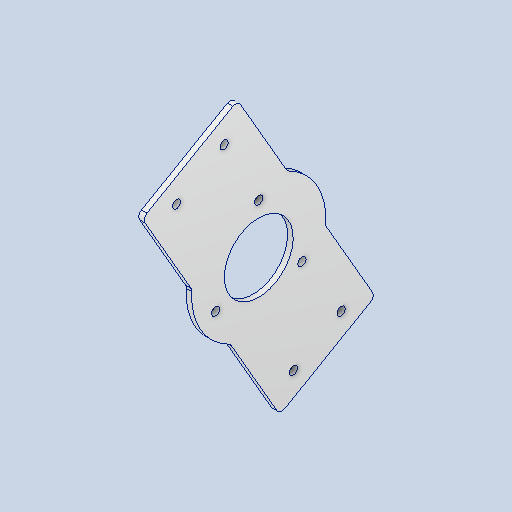
# Autodesk Inventor part: hand-grab-v3-Plate-ASP_F
Saved by Autodesk Inventor 2025.1 (Build 291241000, 241)
## iProperties
Created: 2024-11-30
Part Number: hand-grab-v3-Plate-ASP_F
Material: アルミニウム 6061
Document SubType Name: Modeling
Designer: haruy
Density: 2.7 g/cm^3
Appearance: アルミニウム - フラット
Author: haruy
Autodesk Inventor part; units mm, degrees
ref_plane "YZ Plane" through (0, 0, 0) normal (1, 0, 0) x (0, 1, 0)
ref_plane "XZ Plane" through (0, 0, 0) normal (0, 1, 0) x (-1, 0, 0)
ref_plane "XY Plane" through (0, 0, 0) normal (0, 0, 1) x (1, 0, 0)
sketch "スケッチ1" plane through (0, 0, 0) normal (1, 0, 0) x (0, 1, 0)
  circle A0 centre (73.7666, 7.1685) radius 120
  line L0 (73.7666, 7.1685) -> (-257.6959, 7.1685) construction
  line L1 (141.2666, -109.745) -> (-61.2334, 7.1685)
  circle A1 centre (73.7666, 7.1685) radius 5
  line L2 (73.7666, 7.1685) -> (141.2666, 124.0819) construction
  line L3 (73.7666, 7.1685) -> (141.2666, -109.745) construction
  line L4 (73.7666, 7.1685) -> (-61.2334, 7.1685)
  line L5 (90.8025, 44.6755) -> (85.8025, 36.0153) construction
  line L6 (85.8025, 36.0153) -> (89.2666, 34.0153) construction
  line L7 (89.2666, 34.0153) -> (94.2666, 42.6755) construction
  line L8 (94.2666, 42.6755) -> (90.8025, 44.6755)
  line L9 (94.2666, 42.6755) -> (89.2666, 34.0153) construction
  line L10 (89.2666, 34.0153) -> (92.7307, 32.0153) construction
  line L11 (92.7307, 32.0153) -> (97.7307, 40.6755) construction
  line L12 (97.7307, 40.6755) -> (94.2666, 42.6755)
  line L13 (88.3025, 40.3454) -> (95.2307, 36.3454) construction
  circle A2 centre (73.7666, 7.1685) radius 2.65 construction
  line L14 (90.586, 44.8005) -> (84.086, 33.5422) construction
  line L15 (84.086, 33.5422) -> (79.7559, 36.0422) construction
  line L16 (79.7559, 36.0422) -> (86.2559, 47.3005) construction
  line L17 (86.2559, 47.3005) -> (90.586, 44.8005)
  line L18 (97.9473, 40.5505) -> (91.4473, 29.2922) construction
  line L19 (91.4473, 29.2922) -> (95.7774, 26.7922) construction
  line L20 (95.7774, 26.7922) -> (102.2774, 38.0505) construction
  line L21 (102.2774, 38.0505) -> (97.9473, 40.5505)
  circle A3 centre (73.7666, 7.1685) radius 28.3207 construction
  line L22 (32.7666, 16.4185) -> (32.7666, 11.4185)
  line L23 (32.7666, 11.4185) -> (45.7666, 11.4185) construction
  line L24 (45.7666, 16.4185) -> (32.7666, 16.4185) construction
  line L25 (45.7666, 11.4185) -> (45.7666, 16.4185)
  line L26 (32.7666, 2.9185) -> (45.7666, 2.9185) construction
  line L27 (32.7666, -2.0815) -> (32.7666, 2.9185)
  line L28 (45.7666, -2.0815) -> (32.7666, -2.0815) construction
  line L29 (45.7666, 2.9185) -> (45.7666, -2.0815)
  line L30 (86.2559, -32.9636) -> (90.586, -30.4636)
  line L31 (90.586, -30.4636) -> (84.086, -19.2052) construction
  line L32 (79.7559, -21.7052) -> (86.2559, -32.9636) construction
  line L33 (84.086, -19.2052) -> (79.7559, -21.7052) construction
  line L34 (97.9473, -26.2136) -> (91.4473, -14.9552) construction
  line L35 (102.2774, -23.7136) -> (97.9473, -26.2136)
  line L36 (95.7774, -12.4552) -> (102.2774, -23.7136) construction
  line L37 (91.4473, -14.9552) -> (95.7774, -12.4552) construction
  line L38 (79.7559, 36.0422) -> (79.1397, 34.9748)
  line L39 (95.7774, 26.7922) -> (95.1611, 25.7248) construction
  line L40 (45.7666, 16.4185) -> (46.9991, 16.4185)
  line L41 (45.7666, -2.0815) -> (46.9991, -2.0815)
  line L42 (79.7559, -21.7052) -> (75.9601, -15.1307) construction
  line L43 (95.7774, -12.4552) -> (95.1611, -11.3879) construction
  line L44 (87.3775, 38.7432) -> (77.3775, 21.4227) construction
  line L45 (77.3775, 21.4227) -> (72.1814, 24.4227) construction
  line L46 (72.1814, 24.4227) -> (82.1814, 41.7432) construction
  line L47 (82.1814, 41.7432) -> (87.3775, 38.7432)
  circle A4 centre (77.2795, 27.2529) radius 1.5
  circle A5 centre (82.2795, 35.9131) radius 1.5
  circle A6 centre (89.4038, 20.2529) radius 1.5
  circle A7 centre (94.4038, 28.9131) radius 1.5
  circle A8 centre (44.6166, 14.1685) radius 1.5
  circle A9 centre (54.6166, 14.1685) radius 1.5
  circle A10 centre (54.6166, 0.1685) radius 1.5
  circle A11 centre (44.6166, 0.1685) radius 1.5
  circle A12 centre (82.2795, -21.5762) radius 1.5
  circle A13 centre (77.2795, -12.9159) radius 1.5
  circle A14 centre (89.4038, -5.9159) radius 1.5
  circle A15 centre (94.4038, -14.5762) radius 1.5
  line L48 (74.7795, 22.9227) -> (87.3775, 38.7432) construction
  circle A16 centre (73.7666, 7.1685) radius 34.3835
  line L49 (65.7666, 54.1685) -> (-114.2334, 54.1685) construction
  line L50 (-114.2334, 54.1685) -> (-114.2334, 39.1685)
  line L51 (-114.2334, 39.1685) -> (65.7666, 39.1685) construction
  line L52 (65.7666, 39.1685) -> (65.7666, 54.1685) construction
  circle A17 centre (55.7666, 46.6685) radius 1.5 construction
  circle A18 centre (45.7666, 46.6685) radius 1.5 construction
  line L53 (39.3832, 54.1685) -> (39.3832, 7.1685) construction
  line L54 (65.7666, 54.1685) -> (93.0867, 35.6107) construction
  line L55 (39.3832, -39.8315) -> (39.3832, 7.1685) construction
  line L56 (65.7666, -39.8315) -> (93.0867, -21.2737) construction
  line L57 (65.7666, -39.8315) -> (-114.2334, -39.8315) construction
  line L58 (-114.2334, -24.8315) -> (65.7666, -24.8315) construction
  circle A19 centre (45.7666, -32.3315) radius 1.5 construction
  circle A20 centre (55.7666, -32.3315) radius 1.5 construction
  line L59 (73.7666, 7.1685) -> (56.5749, 36.9454)
  line L60 (65.2352, 41.9454) -> (47.9147, 31.9454)
  line L61 (47.9147, 31.9454) -> (52.9147, 23.2852)
  line L62 (52.9147, 23.2852) -> (70.2352, 33.2852)
  line L63 (70.2352, 33.2852) -> (65.2352, 41.9454)
  circle A21 centre (63.405, 35.1153) radius 1.5
  circle A22 centre (54.7448, 30.1153) radius 1.5
  circle A23 centre (54.7448, -15.7784) radius 1.5
  circle A24 centre (63.405, -20.7784) radius 1.5
  circle A25 centre (103.1501, 2.1685) radius 1.5
  circle A26 centre (103.1501, 12.1685) radius 1.5
  circle A27 centre (73.7666, 7.1685) radius 193.5
  line L64 (-119.0981, 22.835) -> (156.6314, 182.0275)
  line L65 (73.7666, 7.1685) -> (13.7666, 111.0915)
  line L66 (73.7666, 7.1685) -> (73.7666, 200.6685)
  line L67 (127.0679, 14.848) -> (25.5679, 190.6511)
  line L68 (25.5679, 190.6511) -> (12.5775, 183.1511)
  line L69 (12.5775, 183.1511) -> (114.0775, 7.348)
  line L70 (114.0775, 7.348) -> (127.0679, 14.848)
  circle A28 centre (51.8227, 130.1764) radius 1.5
  circle A29 centre (22.8227, 180.4059) radius 1.5
  circle A30 centre (64.6999, 22.8725) radius 1.5
  circle A31 centre (73.7666, 7.1685) radius 12.5
  circle A32 centre (64.6999, -8.5356) radius 1.5
  circle A33 centre (91.9001, 7.1685) radius 1.5
  circle A34 centre (115.5727, 19.7582) radius 1.5
  circle A35 centre (105.5727, 37.0787) radius 1.5
  circle A36 centre (73.7666, 7.1685) radius 24.3835
  line L71 (127.0679, 14.848) -> (95.8462, -3.1779)
  line L72 (107.0679, 49.489) -> (75.8462, 31.4631)
  line L73 (20.4654, -0.511) -> (51.6871, 17.5149)
  circle A37 centre (31.9606, -5.4213) radius 1.5
  circle A38 centre (41.9606, -22.7418) radius 1.5
  line L74 (40.4654, -35.152) -> (-61.0346, 140.6511)
  line L75 (53.4558, -27.652) -> (40.4654, -35.152)
  line L76 (40.4654, -35.152) -> (71.6871, -17.1262)
  point P0 (0, 0)
  point P1 (114.0775, 7.348)
  dimension "d4" = 3
  dimension "d5" = 3
  dimension "d6" = 10
  dimension "d7" = 10
  dimension "d8" = 7.5
  dimension "d9" = 7.5
  dimension "d10" = 60
  dimension "d11" = 10
  dimension "d12" = 10
  dimension "d13" = 10
  dimension "d14" = 3
  dimension "d15" = 5
  dimension "d16" = 5
  dimension "d17" = 360
  dimension "d18" = 387
  dimension "d19" = 110
  dimension "d20" = 60
  dimension "d21" = 15
  dimension "d22" = 73
  dimension "d23" = 3
  dimension "d24" = 3
  dimension "d25" = 7.5
  dimension "d26" = 7.5
  dimension "d27" = 7.5
  dimension "d28" = 7.5
  dimension "d29" = 3
  dimension "d30" = 25
  dimension "d31" = 6.25
  dimension "d32" = 360
  dimension "d33" = 20
  dimension "d34" = 3
  dimension "d35" = 3
  dimension "d36" = 10
  dimension "d37" = 7.5
  dimension "d38" = 7.5
  dimension "d39" = 20
  dimension "d40" = 35
  dimension "d41" = 10
  constraints: 154 end point, 38 centre point, 17 symmetric about line, 8 point on circle, 8 point on line, 6 parallel, 4 perpendicular, 3 coincident, 3 tangent, 1 vertical, 28 other
  measures "d4" diameter of A17
  measures "d5" diameter of A18
  measures "d6" distance from line of A17.centre L52
  measures "d7" distance of A18.centre A17.centre
  measures "d8" distance from line of A17.centre L49
  measures "d9" distance from line of L49 A18.centre
  measures "d11" distance between parallel lines of L60 L62
  measures "d12" distance between parallel lines of L63 L59
  measures "d13" distance between parallel lines of L59 L61
  measures "d14" diameter of A21
  measures "d15" distance from line of L59 A21.centre
  measures "d16" distance from line of A21.centre L60
  measures "d18" diameter of A27
  measures "d19" distance from line of L64 A3.centre
  measures "d21" distance of L68.end L67.end
  measures "d22" distance between parallel lines of L64 L68
  measures "d23" diameter of A28
  measures "d24" diameter of A29
  measures "d25" distance from line of A28.centre L64
  measures "d26" distance from line of A28.centre L69
  measures "d27" distance from line of A29.centre L68
  measures "d28" distance from line of A29.centre L67
  measures "d29" diameter of A30
  measures "d30" diameter of A31
  measures "d31" distance from line of A30.centre L62
  measures "d33" distance from line of L70 point (73.767, 7.168)
  measures "d34" diameter of A34
  measures "d35" diameter of A35
  measures "d36" distance from line of A34.centre L70
  measures "d37" distance from line of L67 A35.centre
  measures "d38" distance from line of L67 A34.centre
  measures "d39" distance of A35.centre A34.centre
  measures "d40" distance from line of L69 point (73.767, 7.168)
  measures "d41" distance from line of L72 A35.centre
extrude "押し出し1" add sketch "スケッチ1" against normal blind 2 contours L67 L70 L69 L72 | A36 L4 A31 L66 | L66 A31 L59 A30 A36 | L69 L71 A16 L72 | L73 A16 L4 | L4 A16 L76 L75 L74 L73 | A16 L71 A25 A36 L72 A5 | L59 A30 A31 L4 A36 | A16 L73 A8 A36 L4 | L4 A36 L76 A24 A16 | A5 L72 | L71 A25 | L73 L25 A8 | A8 L25 L73 | A24 L76 | A11 L29 | L29 A11 | A4 | A6 | A7 | A9 | A10 | A13 | A14 | A23 | A26 picked at (82.8818, 35.0766) picked at (103.6549, 2.1033) picked at (44.5373, 13.2666) picked at (45.8302, 13.5994) picked at (63.236, -21.3216)
fillet "フィレット1" radius 2 8 edges at (-1, 75.8462, 31.4631) (-1, 51.6871, 17.5149) (-1, 20.4654, -0.511) (-1, 40.4654, -35.152) (-1, 71.6871, -17.1262) (-1, 95.8462, -3.1779) (-1, 127.0679, 14.848) (-1, 107.0679, 49.489)
sketch "スケッチ2" plane through (0, 0, 0) normal (1, 0, 0) x (0, 0, -1)
  arc A0 (-47.7569, 108.0679) -> (-48.489, 105.3359) centre (-46.7569, 106.3359) ccw projected
  line L0 (-48.489, 105.3359) -> (-31.7706, 76.3788) projected
  arc A1 (-31.5064, 75.2565) -> (-31.7706, 76.3788) centre (-33.5026, 75.3788) ccw projected
  arc A2 (-31.5064, 75.2565) -> (-18.0471, 51.9444) centre (-7.1685, 73.7666) ccw projected
  arc A3 (-17.2074, 51.1545) -> (-18.0471, 51.9444) centre (-18.9394, 50.1545) ccw projected
  line L1 (-17.2074, 51.1545) -> (-0.489, 22.1974) projected
  arc A4 (-0.489, 22.1974) -> (2.2431, 21.4654) centre (1.2431, 23.1974) ccw projected
  line L2 (2.2431, 21.4654) -> (33.42, 39.4654) projected
  arc A5 (33.42, 39.4654) -> (34.152, 42.1974) centre (32.42, 41.1974) ccw projected
  line L3 (34.152, 42.1974) -> (17.4336, 71.1545) projected
  arc A6 (17.1694, 72.2767) -> (17.4336, 71.1545) centre (19.1657, 72.1545) ccw projected
  arc A7 (17.1694, 72.2767) -> (3.7102, 95.5888) centre (-7.1685, 73.7666) ccw projected
  arc A8 (2.8704, 96.3788) -> (3.7102, 95.5888) centre (4.6025, 97.3788) ccw projected
  line L4 (2.8704, 96.3788) -> (-13.848, 125.3359) projected
  arc A9 (-13.848, 125.3359) -> (-16.58, 126.0679) centre (-15.58, 124.3359) ccw projected
  line L5 (-16.58, 126.0679) -> (-47.7569, 108.0679) projected
  circle A10 centre (-7.1685, 73.7666) radius 12.5 projected
  circle A11 centre (-22.8725, 64.6999) radius 1.5 projected
  circle A12 centre (-37.0787, 105.5727) radius 1.5 projected
  circle A13 centre (-19.7582, 115.5727) radius 1.5 projected
  circle A14 centre (8.5356, 64.6999) radius 1.5 projected
  circle A15 centre (-7.1685, 91.9001) radius 1.5 projected
  circle A16 centre (22.7418, 41.9606) radius 1.5 projected
  circle A17 centre (5.4213, 31.9606) radius 1.5 projected
  point P0 (0, 0)
equation "\"d9\" = d8"
